Autodesk Inventor part; units mm, degrees
(part 2 of 3)
  spline S148 degree 2 poles (-84.7647, -63.9255) (-84.6572, -63.7642) (-84.2951, -63.5775) (-84.0744, -63.5775) knots 0 0 0 1 2 2 2
  spline S149 degree 2 poles (-84.0744, -63.5775) (-83.6641, -63.5775) (-83.2227, -64.1263) (-83.2227, -64.6554) knots 0 0 0 1 2 2 2
  spline S150 degree 2 poles (-84.1423, -64.6809) (-84.1423, -64.463) (-84.3092, -64.2423) (-84.4676, -64.2423) knots 0 0 0 1 2 2 2
  spline S151 degree 2 poles (-84.4676, -64.2423) (-84.6063, -64.2423) (-84.7902, -64.4743) (-84.7902, -64.6583) knots 0 0 0 1 2 2 2
  line L119 (-84.7902, -64.6583) -> (-84.7902, -64.7912)
  spline S152 degree 2 poles (-84.7902, -64.7912) (-84.7902, -64.978) (-84.6233, -65.1987) (-84.4846, -65.1987) knots 0 0 0 1 2 2 2
  spline S153 degree 2 poles (-84.4846, -65.1987) (-84.3205, -65.1987) (-84.1423, -64.9299) (-84.1423, -64.6809) knots 0 0 0 1 2 2 2
  spline S154 degree 2 poles (-82.4588, -66.834) (-82.5862, -66.834) (-82.8776, -66.7887) (-82.9936, -66.7463) knots 0 0 0 1 2 2 2
  line L120 (-82.9936, -66.7463) -> (-82.9936, -66.0644)
  spline S155 degree 2 poles (-82.9936, -66.0644) (-82.9398, -66.104) (-82.7304, -66.1719) (-82.6371, -66.1719) knots 0 0 0 1 2 2 2
  spline S156 degree 2 poles (-82.6371, -66.1719) (-82.3824, -66.1719) (-82.3004, -65.9711) knots 0 0 0 1 1 1
  line L121 (-82.3004, -65.9711) -> (-82.2297, -65.8013)
  line L122 (-82.2297, -65.8013) -> (-83.1407, -63.6312)
  line L123 (-83.1407, -63.6312) -> (-82.1391, -63.6312)
  line L124 (-82.1391, -63.6312) -> (-81.876, -64.6809)
  spline S157 degree 2 poles (-81.876, -64.6809) (-81.7996, -64.9751) (-81.7911, -65.077) knots 0 0 0 1 1 1
  line L125 (-81.7911, -65.077) -> (-81.7826, -65.077)
  spline S158 degree 2 poles (-81.7826, -65.077) (-81.777, -65.0289) (-81.7543, -64.9157) (-81.4346, -63.6312) knots 0 0 0 1 2 2 2
  line L126 (-81.4346, -63.6312) -> (-80.5547, -63.6312)
  line L127 (-80.5547, -63.6312) -> (-81.3554, -65.872)
  spline S159 degree 2 poles (-81.3554, -65.872) (-81.5365, -66.387) (-82.0712, -66.834) (-82.4588, -66.834) knots 0 0 0 1 2 2 2
  spline S160 degree 2 poles (-79.3947, -65.4307) (-79.3947, -65.6259) (-79.6663, -65.8635) (-79.9068, -65.8635) knots 0 0 0 1 2 2 2
  spline S161 degree 2 poles (-79.9068, -65.8635) (-80.1275, -65.8635) (-80.4048, -65.6146) (-80.4048, -65.4307) knots 0 0 0 1 2 2 2
  spline S162 degree 2 poles (-80.4048, -65.4307) (-80.4048, -65.2439) (-80.1303, -65.0119) (-79.8983, -65.0119) knots 0 0 0 1 2 2 2
  spline S163 degree 2 poles (-79.8983, -65.0119) (-79.672, -65.0119) (-79.3947, -65.2439) (-79.3947, -65.4307) knots 0 0 0 1 2 2 2
  spline S164 degree 2 poles (-79.3947, -64.05) (-79.3947, -64.2452) (-79.6691, -64.48) (-79.9068, -64.48) knots 0 0 0 1 2 2 2
  spline S165 degree 2 poles (-79.9068, -64.48) (-80.1246, -64.48) (-80.4048, -64.2339) (-80.4048, -64.05) knots 0 0 0 1 2 2 2
  spline S166 degree 2 poles (-80.4048, -64.05) (-80.4048, -63.8632) (-80.1303, -63.6312) (-79.8983, -63.6312) knots 0 0 0 1 2 2 2
  spline S167 degree 2 poles (-79.8983, -63.6312) (-79.672, -63.6312) (-79.3947, -63.8632) (-79.3947, -64.05) knots 0 0 0 1 2 2 2
  spline S168 degree 2 poles (-137.9162, -70.7081) (-137.9162, -70.8722) (-138.086, -71.1636) (-138.3774, -71.3305) (-138.5387, -71.3305) knots 0 0 0 1 2 3 3 3
  spline S169 degree 2 poles (-138.5387, -71.3305) (-138.7905, -71.3305) (-139.1526, -70.9684) (-139.1526, -70.7081) knots 0 0 0 1 2 2 2
  spline S170 degree 2 poles (-139.1526, -70.7081) (-139.1526, -70.4563) (-138.7961, -70.0941) (-138.5387, -70.0941) knots 0 0 0 1 2 2 2
  spline S171 degree 2 poles (-138.5387, -70.0941) (-138.2755, -70.0941) (-137.9162, -70.4619) (-137.9162, -70.7081) knots 0 0 0 1 2 2 2
  line L128 (-128.1268, -71.7464) -> (-128.2598, -71.1862)
  line L129 (-128.2598, -71.1862) -> (-129.1708, -71.1862)
  line L130 (-129.1708, -71.1862) -> (-129.3151, -71.7464)
  line L131 (-129.3151, -71.7464) -> (-130.3082, -71.7464)
  line L132 (-130.3082, -71.7464) -> (-129.2585, -68.6964)
  line L133 (-129.2585, -68.6964) -> (-128.1183, -68.6964)
  line L134 (-128.1183, -68.6964) -> (-127.128, -71.7464)
  line L135 (-127.128, -71.7464) -> (-128.1268, -71.7464)
  line L136 (-128.704, -69.3613) -> (-128.7238, -69.3613)
  spline S172 degree 2 poles (-128.7238, -69.3613) (-128.7294, -69.4123) (-128.7804, -69.6471) (-129.0124, -70.5327) knots 0 0 0 1 2 2 2
  line L137 (-129.0124, -70.5327) -> (-128.4295, -70.5327)
  line L138 (-128.4295, -70.5327) -> (-128.6417, -69.7037)
  spline S173 degree 2 poles (-128.6417, -69.7037) (-128.687, -69.5198) (-128.704, -69.3613) knots 0 0 0 1 1 1
  line L139 (-126.8536, -71.7464) -> (-126.8536, -68.521)
  line L140 (-126.8536, -68.521) -> (-125.9482, -68.521)
  line L141 (-125.9482, -68.521) -> (-125.9482, -71.7464)
  line L142 (-125.9482, -71.7464) -> (-126.8536, -71.7464)
  spline S174 degree 2 poles (-123.8347, -69.1803) (-123.9762, -69.1322) (-124.095, -69.1322) knots 0 0 0 1 1 1
  spline S175 degree 2 poles (-124.095, -69.1322) (-124.2478, -69.1322) (-124.3921, -69.2878) (-124.3921, -69.4179) knots 0 0 0 1 2 2 2
  line L143 (-124.3921, -69.4179) -> (-124.3921, -69.5679)
  line L144 (-124.3921, -69.5679) -> (-123.8885, -69.5679)
  line L145 (-123.8885, -69.5679) -> (-123.8885, -70.196)
  line L146 (-123.8885, -70.196) -> (-124.3921, -70.196)
  line L147 (-124.3921, -70.196) -> (-124.3921, -71.7464)
  line L148 (-124.3921, -71.7464) -> (-125.2975, -71.7464)
  line L149 (-125.2975, -71.7464) -> (-125.2975, -70.196)
  line L150 (-125.2975, -70.196) -> (-125.6625, -70.196)
  line L151 (-125.6625, -70.196) -> (-125.6625, -69.5679)
  line L152 (-125.6625, -69.5679) -> (-125.2975, -69.5679)
  line L153 (-125.2975, -69.5679) -> (-125.2975, -69.367)
  spline S176 degree 2 poles (-125.2975, -69.367) (-125.2975, -69.101) (-125.0513, -68.6964) (-124.5817, -68.4701) (-124.245, -68.4701) knots 0 0 0 1 2 3 3 3
  spline S177 degree 2 poles (-124.245, -68.4701) (-124.0016, -68.4701) (-123.8347, -68.5182) knots 0 0 0 1 1 1
  line L154 (-123.8347, -68.5182) -> (-123.8347, -69.1803)
  line L155 (-122.4257, -71.7464) -> (-122.4257, -71.4154)
  line L156 (-122.4257, -71.4154) -> (-122.4342, -71.4154)
  spline S178 degree 2 poles (-122.4342, -71.4154) (-122.6521, -71.8002) (-123.0991, -71.8002) knots 0 0 0 1 1 1
  spline S179 degree 2 poles (-123.0991, -71.8002) (-123.4075, -71.8002) (-123.7555, -71.4352) (-123.7555, -71.1268) knots 0 0 0 1 2 2 2
  spline S180 degree 2 poles (-123.7555, -71.1268) (-123.7555, -70.4846) (-122.9661, -70.3827) knots 0 0 0 1 1 1
  line L157 (-122.9661, -70.3827) -> (-122.4257, -70.312)
  spline S181 degree 2 poles (-122.4257, -70.312) (-122.4257, -70.2045) (-122.6181, -70.0687) (-122.7794, -70.0687) knots 0 0 0 1 2 2 2
  spline S182 degree 2 poles (-122.7794, -70.0687) (-123.1444, -70.0687) (-123.5518, -70.278) knots 0 0 0 1 1 1
  line L158 (-123.5518, -70.278) -> (-123.5518, -69.6895)
  spline S183 degree 2 poles (-123.5518, -69.6895) (-123.3764, -69.6131) (-122.8416, -69.5141) (-122.6521, -69.5141) knots 0 0 0 1 2 2 2
  spline S184 degree 2 poles (-122.6521, -69.5141) (-122.0975, -69.5141) (-121.5967, -69.9894) (-121.5967, -70.544) knots 0 0 0 1 2 2 2
  line L159 (-121.5967, -70.544) -> (-121.5967, -71.7464)
  line L160 (-121.5967, -71.7464) -> (-122.4257, -71.7464)
  spline S185 degree 2 poles (-122.9633, -71.0052) (-122.9633, -71.0929) (-122.8501, -71.2089) (-122.7454, -71.2089) knots 0 0 0 1 2 2 2
  spline S186 degree 2 poles (-122.7454, -71.2089) (-122.604, -71.2089) (-122.4257, -70.9967) (-122.4257, -70.8298) knots 0 0 0 1 2 2 2
  line L161 (-122.4257, -70.8298) -> (-122.4257, -70.7477)
  line L162 (-122.4257, -70.7477) -> (-122.7341, -70.7901)
  spline S187 degree 2 poles (-122.7341, -70.7901) (-122.9633, -70.8298) (-122.9633, -71.0052) knots 0 0 0 1 1 1
  line L163 (-119.7775, -71.7464) -> (-119.7775, -70.5581)
  spline S188 degree 2 poles (-119.7775, -70.5581) (-119.7775, -70.3544) (-119.8991, -70.179) (-120.0349, -70.179) knots 0 0 0 1 2 2 2
  spline S189 degree 2 poles (-120.0349, -70.179) (-120.1509, -70.179) (-120.2839, -70.3629) (-120.2839, -70.5044) knots 0 0 0 1 2 2 2
  line L164 (-120.2839, -70.5044) -> (-120.2839, -71.7464)
  line L165 (-120.2839, -71.7464) -> (-121.1893, -71.7464)
  line L166 (-121.1893, -71.7464) -> (-121.1893, -69.5679)
  line L167 (-121.1893, -69.5679) -> (-120.2839, -69.5679)
  line L168 (-120.2839, -69.5679) -> (-120.2839, -69.9074)
  line L169 (-120.2839, -69.9074) -> (-120.2754, -69.9074)
  spline S190 degree 2 poles (-120.2754, -69.9074) (-120.1679, -69.7207) (-119.8001, -69.5141) (-119.5851, -69.5141) knots 0 0 0 1 2 2 2
  spline S191 degree 2 poles (-119.5851, -69.5141) (-118.8721, -69.5141) (-118.8721, -70.4167) knots 0 0 0 1 1 1
  line L170 (-118.8721, -70.4167) -> (-118.8721, -71.7464)
  line L171 (-118.8721, -71.7464) -> (-119.7775, -71.7464)
  spline S192 degree 2 poles (-116.04, -70.6176) (-116.04, -71.1693) (-116.7048, -71.8002) (-117.3018, -71.8002) knots 0 0 0 1 2 2 2
  spline S193 degree 2 poles (-117.3018, -71.8002) (-117.896, -71.8002) (-118.558, -71.1862) (-118.558, -70.643) knots 0 0 0 1 2 2 2
  spline S194 degree 2 poles (-118.558, -70.643) (-118.558, -70.2978) (-118.2468, -69.7857) (-117.6725, -69.5141) (-117.299, -69.5141) knots 0 0 0 1 2 3 3 3
  spline S195 degree 2 poles (-117.299, -69.5141) (-116.9114, -69.5141) (-116.3427, -69.7999) (-116.04, -70.3063) (-116.04, -70.6176) knots 0 0 0 1 2 3 3 3
  spline S196 degree 2 poles (-116.9595, -70.6232) (-116.9595, -70.179) (-117.299, -70.179) knots 0 0 0 1 1 1
  spline S197 degree 2 poles (-117.299, -70.179) (-117.6385, -70.179) (-117.6385, -70.643) knots 0 0 0 1 1 1
  spline S198 degree 2 poles (-117.6385, -70.643) (-117.6385, -71.1353) (-117.2933, -71.1353) knots 0 0 0 1 1 1
  spline S199 degree 2 poles (-117.2933, -71.1353) (-116.9595, -71.1353) (-116.9595, -70.6232) knots 0 0 0 1 1 1
  line L172 (-114.4074, -71.7464) -> (-114.4074, -68.6964)
  line L173 (-114.4074, -68.6964) -> (-112.509, -68.6964)
  line L174 (-112.509, -68.6964) -> (-112.509, -69.4151)
  line L175 (-112.509, -69.4151) -> (-113.4879, -69.4151)
  line L176 (-113.4879, -69.4151) -> (-113.4879, -69.8593)
  line L177 (-113.4879, -69.8593) -> (-112.5684, -69.8593)
  line L178 (-112.5684, -69.8593) -> (-112.5684, -70.5779)
  line L179 (-112.5684, -70.5779) -> (-113.4879, -70.5779)
  line L180 (-113.4879, -70.5779) -> (-113.4879, -71.0278)
  line L181 (-113.4879, -71.0278) -> (-112.4382, -71.0278)
  line L182 (-112.4382, -71.0278) -> (-112.4382, -71.7464)
  line L183 (-112.4382, -71.7464) -> (-114.4074, -71.7464)
  line L184 (-109.2609, -71.7464) -> (-109.2609, -70.4902)
  spline S200 degree 2 poles (-109.2609, -70.4902) (-109.2609, -70.3346) (-109.3741, -70.179) (-109.5014, -70.179) knots 0 0 0 1 2 2 2
  spline S201 degree 2 poles (-109.5014, -70.179) (-109.6259, -70.179) (-109.7674, -70.3686) (-109.7674, -70.5355) knots 0 0 0 1 2 2 2
  line L185 (-109.7674, -70.5355) -> (-109.7674, -71.7464)
  line L186 (-109.7674, -71.7464) -> (-110.6727, -71.7464)
  line L187 (-110.6727, -71.7464) -> (-110.6727, -70.5129)
  spline S202 degree 2 poles (-110.6727, -70.5129) (-110.6727, -70.179) (-110.8991, -70.179) knots 0 0 0 1 1 1
  spline S203 degree 2 poles (-110.8991, -70.179) (-111.0377, -70.179) (-111.1792, -70.3714) (-111.1792, -70.5525) knots 0 0 0 1 2 2 2
  line L188 (-111.1792, -70.5525) -> (-111.1792, -71.7464)
  line L189 (-111.1792, -71.7464) -> (-112.0846, -71.7464)
  line L190 (-112.0846, -71.7464) -> (-112.0846, -69.5679)
  line L191 (-112.0846, -69.5679) -> (-111.1792, -69.5679)
  line L192 (-111.1792, -69.5679) -> (-111.1792, -69.9131)
  line L193 (-111.1792, -69.9131) -> (-111.1707, -69.9131)
  spline S204 degree 2 poles (-111.1707, -69.9131) (-111.1198, -69.8225) (-110.8963, -69.6301) (-110.6162, -69.5141) (-110.4521, -69.5141) knots 0 0 0 1 2 3 3 3
  spline S205 degree 2 poles (-110.4521, -69.5141) (-110.2201, -69.5141) (-109.9032, -69.698) (-109.7985, -69.8961) knots 0 0 0 1 2 2 2
  spline S206 degree 2 poles (-109.7985, -69.8961) (-109.6825, -69.7122) (-109.2977, -69.5141) (-109.0657, -69.5141) knots 0 0 0 1 2 2 2
  spline S207 degree 2 poles (-109.0657, -69.5141) (-108.7205, -69.5141) (-108.3555, -69.9612) (-108.3555, -70.3827) knots 0 0 0 1 2 2 2
  line L194 (-108.3555, -70.3827) -> (-108.3555, -71.7464)
  line L195 (-108.3555, -71.7464) -> (-109.2609, -71.7464)
  line L196 (-106.7372, -71.7464) -> (-106.7372, -71.4154)
  line L197 (-106.7372, -71.4154) -> (-106.7457, -71.4154)
  spline S208 degree 2 poles (-106.7457, -71.4154) (-106.9635, -71.8002) (-107.4106, -71.8002) knots 0 0 0 1 1 1
  spline S209 degree 2 poles (-107.4106, -71.8002) (-107.7189, -71.8002) (-108.067, -71.4352) (-108.067, -71.1268) knots 0 0 0 1 2 2 2
  spline S210 degree 2 poles (-108.067, -71.1268) (-108.067, -70.4846) (-107.2776, -70.3827) knots 0 0 0 1 1 1
  line L198 (-107.2776, -70.3827) -> (-106.7372, -70.312)
  spline S211 degree 2 poles (-106.7372, -70.312) (-106.7372, -70.2045) (-106.9296, -70.0687) (-107.0908, -70.0687) knots 0 0 0 1 2 2 2
  spline S212 degree 2 poles (-107.0908, -70.0687) (-107.4558, -70.0687) (-107.8632, -70.278) knots 0 0 0 1 1 1
  line L199 (-107.8632, -70.278) -> (-107.8632, -69.6895)
  spline S213 degree 2 poles (-107.8632, -69.6895) (-107.6878, -69.6131) (-107.1531, -69.5141) (-106.9635, -69.5141) knots 0 0 0 1 2 2 2
  spline S214 degree 2 poles (-106.9635, -69.5141) (-106.409, -69.5141) (-105.9082, -69.9894) (-105.9082, -70.544) knots 0 0 0 1 2 2 2
  line L200 (-105.9082, -70.544) -> (-105.9082, -71.7464)
  line L201 (-105.9082, -71.7464) -> (-106.7372, -71.7464)
  spline S215 degree 2 poles (-107.2747, -71.0052) (-107.2747, -71.0929) (-107.1616, -71.2089) (-107.0569, -71.2089) knots 0 0 0 1 2 2 2
  spline S216 degree 2 poles (-107.0569, -71.2089) (-106.9154, -71.2089) (-106.7372, -70.9967) (-106.7372, -70.8298) knots 0 0 0 1 2 2 2
  line L202 (-106.7372, -70.8298) -> (-106.7372, -70.7477)
  line L203 (-106.7372, -70.7477) -> (-107.0456, -70.7901)
  spline S217 degree 2 poles (-107.0456, -70.7901) (-107.2747, -70.8298) (-107.2747, -71.0052) knots 0 0 0 1 1 1
  line L204 (-104.0889, -71.7464) -> (-104.0889, -70.5581)
  spline S218 degree 2 poles (-104.0889, -70.5581) (-104.0889, -70.3544) (-104.2106, -70.179) (-104.3464, -70.179) knots 0 0 0 1 2 2 2
  spline S219 degree 2 poles (-104.3464, -70.179) (-104.4624, -70.179) (-104.5954, -70.3629) (-104.5954, -70.5044) knots 0 0 0 1 2 2 2
  line L205 (-104.5954, -70.5044) -> (-104.5954, -71.7464)
  line L206 (-104.5954, -71.7464) -> (-105.5008, -71.7464)
  line L207 (-105.5008, -71.7464) -> (-105.5008, -69.5679)
  line L208 (-105.5008, -69.5679) -> (-104.5954, -69.5679)
  line L209 (-104.5954, -69.5679) -> (-104.5954, -69.9074)
  line L210 (-104.5954, -69.9074) -> (-104.5869, -69.9074)
  spline S220 degree 2 poles (-104.5869, -69.9074) (-104.4794, -69.7207) (-104.1116, -69.5141) (-103.8965, -69.5141) knots 0 0 0 1 2 2 2
  spline S221 degree 2 poles (-103.8965, -69.5141) (-103.1836, -69.5141) (-103.1836, -70.4167) knots 0 0 0 1 1 1
  line L211 (-103.1836, -70.4167) -> (-103.1836, -71.7464)
  line L212 (-103.1836, -71.7464) -> (-104.0889, -71.7464)
  line L213 (-101.3869, -71.7464) -> (-101.3869, -71.4098)
  line L214 (-101.3869, -71.4098) -> (-101.3954, -71.4098)
  spline S222 degree 2 poles (-101.3954, -71.4098) (-101.5086, -71.5654) (-101.6897, -71.7097) (-101.916, -71.8002) (-102.066, -71.8002) knots 0 0 0 1 2 3 3 3
  spline S223 degree 2 poles (-102.066, -71.8002) (-102.4253, -71.8002) (-102.7988, -71.3362) (-102.7988, -70.8835) knots 0 0 0 1 2 2 2
  line L215 (-102.7988, -70.8835) -> (-102.7988, -69.5679)
  line L216 (-102.7988, -69.5679) -> (-101.8934, -69.5679)
  line L217 (-101.8934, -69.5679) -> (-101.8934, -70.8128)
  spline S224 degree 2 poles (-101.8934, -70.8128) (-101.8934, -71.1353) (-101.6529, -71.1353) knots 0 0 0 1 1 1
  spline S225 degree 2 poles (-101.6529, -71.1353) (-101.5199, -71.1353) (-101.3869, -70.9599) (-101.3869, -70.8015) knots 0 0 0 1 2 2 2
  line L218 (-101.3869, -70.8015) -> (-101.3869, -69.5679)
  line L219 (-101.3869, -69.5679) -> (-100.4816, -69.5679)
  line L220 (-100.4816, -69.5679) -> (-100.4816, -71.7464)
  line L221 (-100.4816, -71.7464) -> (-101.3869, -71.7464)
  spline S226 degree 2 poles (-99.265, -70.9146) (-99.2423, -71.0561) (-98.965, -71.2145) (-98.7387, -71.2145) knots 0 0 0 1 2 2 2
  spline S227 degree 2 poles (-98.7387, -71.2145) (-98.4218, -71.2145) (-98.1389, -71.0929) knots 0 0 0 1 1 1
  line L222 (-98.1389, -71.0929) -> (-98.1389, -71.6672)
  spline S228 degree 2 poles (-98.1389, -71.6672) (-98.4671, -71.8002) (-98.9396, -71.8002) knots 0 0 0 1 1 1
  spline S229 degree 2 poles (-98.9396, -71.8002) (-99.5083, -71.8002) (-100.142, -71.2174) (-100.142, -70.7053) knots 0 0 0 1 2 2 2
  spline S230 degree 2 poles (-100.142, -70.7053) (-100.142, -70.3544) (-99.8648, -69.8197) (-99.3187, -69.5141) (-98.9877, -69.5141) knots 0 0 0 1 2 3 3 3
  spline S231 degree 2 poles (-98.9877, -69.5141) (-98.651, -69.5141) (-98.17, -69.7772) (-97.921, -70.2554) (-97.921, -70.5751) knots 0 0 0 1 2 3 3 3
  line L223 (-97.921, -70.5751) -> (-97.921, -70.9146)
  line L224 (-97.921, -70.9146) -> (-99.265, -70.9146)
  spline S232 degree 2 poles (-98.7217, -70.4393) (-98.7217, -70.063) (-98.9905, -70.063) knots 0 0 0 1 1 1
  spline S233 degree 2 poles (-98.9905, -70.063) (-99.1037, -70.063) (-99.2565, -70.2695) (-99.2706, -70.4393) knots 0 0 0 1 2 2 2
  line L225 (-99.2706, -70.4393) -> (-98.7217, -70.4393)
  line L226 (-97.607, -71.7464) -> (-97.607, -68.521)
  line L227 (-97.607, -68.521) -> (-96.7016, -68.521)
  line L228 (-96.7016, -68.521) -> (-96.7016, -71.7464)
  line L229 (-96.7016, -71.7464) -> (-97.607, -71.7464)
  spline S234 degree 2 poles (-95.485, -70.9146) (-95.4624, -71.0561) (-95.1851, -71.2145) (-94.9587, -71.2145) knots 0 0 0 1 2 2 2
  spline S235 degree 2 poles (-94.9587, -71.2145) (-94.6419, -71.2145) (-94.3589, -71.0929) knots 0 0 0 1 1 1
  line L230 (-94.3589, -71.0929) -> (-94.3589, -71.6672)
  spline S236 degree 2 poles (-94.3589, -71.6672) (-94.6871, -71.8002) (-95.1596, -71.8002) knots 0 0 0 1 1 1
  spline S237 degree 2 poles (-95.1596, -71.8002) (-95.7283, -71.8002) (-96.3621, -71.2174) (-96.3621, -70.7053) knots 0 0 0 1 2 2 2
  spline S238 degree 2 poles (-96.3621, -70.7053) (-96.3621, -70.3544) (-96.0848, -69.8197) (-95.5388, -69.5141) (-95.2077, -69.5141) knots 0 0 0 1 2 3 3 3
  spline S239 degree 2 poles (-95.2077, -69.5141) (-94.871, -69.5141) (-94.39, -69.7772) (-94.1411, -70.2554) (-94.1411, -70.5751) knots 0 0 0 1 2 3 3 3
  line L231 (-94.1411, -70.5751) -> (-94.1411, -70.9146)
  line L232 (-94.1411, -70.9146) -> (-95.485, -70.9146)
  spline S240 degree 2 poles (-94.9418, -70.4393) (-94.9418, -70.063) (-95.2106, -70.063) knots 0 0 0 1 1 1
  spline S241 degree 2 poles (-95.2106, -70.063) (-95.3237, -70.063) (-95.4765, -70.2695) (-95.4907, -70.4393) knots 0 0 0 1 2 2 2
  line L233 (-95.4907, -70.4393) -> (-94.9418, -70.4393)
  spline S242 degree 2 poles (-24.5942, -53.8935) (-24.5942, -54.289) (-24.8759, -55.0008) (-25.128, -55.248) knots 0 0 0 1 2 2 2
  spline S243 degree 2 poles (-25.128, -55.248) (-25.4444, -55.5594) (-26.2996, -55.8807) (-26.9521, -55.8807) knots 0 0 0 1 2 2 2
  line L234 (-26.9521, -55.8807) -> (-27.6392, -55.8807)
  line L235 (-27.6392, -55.8807) -> (-27.6392, -58.1546)
  line L236 (-27.6392, -58.1546) -> (-28.4499, -58.1546)
  line L237 (-28.4499, -58.1546) -> (-28.4499, -52.0546)
  line L238 (-28.4499, -52.0546) -> (-26.9175, -52.0546)
  spline S244 degree 2 poles (-26.9175, -52.0546) (-26.3737, -52.0546) (-25.6125, -52.2326) (-25.3208, -52.4353) knots 0 0 0 1 2 2 2
  spline S245 degree 2 poles (-25.3208, -52.4353) (-24.9797, -52.6676) (-24.5942, -53.3844) (-24.5942, -53.8935) knots 0 0 0 1 2 2 2
  spline S246 degree 2 poles (-25.4395, -53.9182) (-25.4395, -53.6019) (-25.657, -53.1372) (-25.8794, -52.9889) knots 0 0 0 1 2 2 2
  spline S247 degree 2 poles (-25.8794, -52.9889) (-26.0722, -52.8604) (-26.5863, -52.7566) (-26.9669, -52.7566) knots 0 0 0 1 2 2 2
  line L239 (-26.9669, -52.7566) -> (-27.6392, -52.7566)
  line L240 (-27.6392, -52.7566) -> (-27.6392, -55.1887)
  line L241 (-27.6392, -55.1887) -> (-27.0856, -55.1887)
  spline S248 degree 2 poles (-27.0856, -55.1887) (-26.5913, -55.1887) (-25.9832, -55.0305) (-25.7855, -54.8229) knots 0 0 0 1 2 2 2
  spline S249 degree 2 poles (-25.7855, -54.8229) (-25.6026, -54.64) (-25.4395, -54.2099) (-25.4395, -53.9182) knots 0 0 0 1 2 2 2
  line L242 (-21.4552, -54.4027) -> (-21.4947, -54.4027)
  spline S250 degree 2 poles (-21.4947, -54.4027) (-21.5837, -54.378) (-21.7765, -54.3681) (-21.91, -54.3681) knots 0 0 0 1 2 2 2
  spline S251 degree 2 poles (-21.91, -54.3681) (-22.2214, -54.3681) (-22.8344, -54.64) (-23.1112, -54.9069) knots 0 0 0 1 2 2 2
  line L243 (-23.1112, -54.9069) -> (-23.1112, -58.1546)
  line L244 (-23.1112, -58.1546) -> (-23.8823, -58.1546)
  line L245 (-23.8823, -58.1546) -> (-23.8823, -53.5772)
  line L246 (-23.8823, -53.5772) -> (-23.1112, -53.5772)
  line L247 (-23.1112, -53.5772) -> (-23.1112, -54.2593)
  spline S252 degree 2 poles (-23.1112, -54.2593) (-22.691, -53.8836) (-22.0632, -53.5772) (-21.7666, -53.5772) knots 0 0 0 1 2 2 2
  spline S253 degree 2 poles (-21.7666, -53.5772) (-21.648, -53.5772) (-21.5293, -53.587) (-21.4552, -53.6019) knots 0 0 0 1 2 2 2
  line L248 (-21.4552, -53.6019) -> (-21.4552, -54.4027)
  spline S254 degree 2 poles (-17.0952, -55.8659) (-17.0952, -57.0226) (-18.2075, -58.2832) (-19.1368, -58.2832) knots 0 0 0 1 2 2 2
  spline S255 degree 2 poles (-19.1368, -58.2832) (-20.0908, -58.2832) (-21.1833, -56.9831) (-21.1833, -55.8659) knots 0 0 0 1 2 2 2
  spline S256 degree 2 poles (-21.1833, -55.8659) (-21.1833, -54.7191) (-20.0562, -53.4486) (-19.1368, -53.4486) knots 0 0 0 1 2 2 2
  spline S257 degree 2 poles (-19.1368, -53.4486) (-18.2075, -53.4486) (-17.0952, -54.7141) (-17.0952, -55.8659) knots 0 0 0 1 2 2 2
  spline S258 degree 2 poles (-17.8911, -55.8659) (-17.8911, -54.9761) (-18.5387, -54.111) (-19.1368, -54.111) knots 0 0 0 1 2 2 2
  spline S259 degree 2 poles (-19.1368, -54.111) (-19.7349, -54.111) (-20.3874, -54.9761) (-20.3874, -55.8659) knots 0 0 0 1 2 2 2
  spline S260 degree 2 poles (-20.3874, -55.8659) (-20.3874, -56.731) (-19.7349, -57.6208) (-19.1368, -57.6208) knots 0 0 0 1 2 2 2
  spline S261 degree 2 poles (-19.1368, -57.6208) (-18.5436, -57.6208) (-17.8911, -56.7458) (-17.8911, -55.8659) knots 0 0 0 1 2 2 2
  spline S262 degree 2 poles (-16.1412, -58.8862) (-16.0621, -58.9208) (-15.7605, -59.0296) (-15.5677, -59.0741) knots 0 0 0 1 2 2 2
  spline S263 degree 2 poles (-15.5677, -59.0741) (-15.3552, -59.1285) (-14.9943, -59.1927) (-14.7818, -59.1927) knots 0 0 0 1 2 2 2
  spline S264 degree 2 poles (-14.7818, -59.1927) (-14.4259, -59.1927) (-13.9315, -59.0049) (-13.7931, -58.8368) knots 0 0 0 1 2 2 2
  spline S265 degree 2 poles (-13.7931, -58.8368) (-13.6596, -58.6687) (-13.5558, -58.2288) (-13.5558, -57.947) knots 0 0 0 1 2 2 2
  line L249 (-13.5558, -57.947) -> (-13.5558, -57.5466)
  spline S266 degree 2 poles (-13.5558, -57.5466) (-13.8673, -57.8185) (-14.4654, -58.0755) (-14.9152, -58.0755) knots 0 0 0 1 2 2 2
  spline S267 degree 2 poles (-14.9152, -58.0755) (-15.6963, -58.0755) (-16.6207, -56.9139) (-16.6207, -55.8214) knots 0 0 0 1 2 2 2
  spline S268 degree 2 poles (-16.6207, -55.8214) (-16.6207, -55.2529) (-16.2994, -54.373) (-16.0324, -54.0616) knots 0 0 0 1 2 2 2
  spline S269 degree 2 poles (-16.0324, -54.0616) (-15.7754, -53.7699) (-15.0685, -53.4486) (-14.6928, -53.4486) knots 0 0 0 1 2 2 2
  spline S270 degree 2 poles (-14.6928, -53.4486) (-14.3369, -53.4486) (-13.8178, -53.6167) (-13.5558, -53.7699) knots 0 0 0 1 2 2 2
  line L250 (-13.5558, -53.7699) -> (-13.5113, -53.5772)
  line L251 (-13.5113, -53.5772) -> (-12.7847, -53.5772)
  line L252 (-12.7847, -53.5772) -> (-12.7847, -57.6306)
  spline S271 degree 2 poles (-12.7847, -57.6306) (-12.7847, -58.7973) (-13.7981, -59.8848) (-14.8411, -59.8848) knots 0 0 0 1 2 2 2
  spline S272 degree 2 poles (-14.8411, -59.8848) (-15.1772, -59.8848) (-15.8792, -59.776) (-16.1807, -59.687) knots 0 0 0 1 2 2 2
  line L253 (-16.1807, -59.687) -> (-16.1807, -58.8862)
  line L254 (-16.1807, -58.8862) -> (-16.1412, -58.8862)
  line L255 (-13.5558, -56.9139) -> (-13.5558, -54.3977)
  spline S273 degree 2 poles (-13.5558, -54.3977) (-13.8425, -54.2593) (-14.327, -54.1407) (-14.5692, -54.1407) knots 0 0 0 1 2 2 2
  spline S274 degree 2 poles (-14.5692, -54.1407) (-15.1525, -54.1407) (-15.8248, -55.0008) (-15.8248, -55.8066) knots 0 0 0 1 2 2 2
  spline S275 degree 2 poles (-15.8248, -55.8066) (-15.8248, -56.5678) (-15.3156, -57.3637) (-14.7422, -57.3637) knots 0 0 0 1 2 2 2
  spline S276 degree 2 poles (-14.7422, -57.3637) (-14.4407, -57.3637) (-13.8079, -57.1264) (-13.5558, -56.9139) knots 0 0 0 1 2 2 2
  spline S277 degree 2 poles (-9.6803, -58.2584) (-10.7777, -58.2584) (-11.9839, -57.0276) (-11.9839, -55.8906) knots 0 0 0 1 2 2 2
  spline S278 degree 2 poles (-11.9839, -55.8906) (-11.9839, -54.7734) (-10.8123, -53.4486) (-9.8682, -53.4486) knots 0 0 0 1 2 2 2
  spline S279 degree 2 poles (-9.8682, -53.4486) (-9.443, -53.4486) (-8.7856, -53.6958) (-8.5434, -53.9578) knots 0 0 0 1 2 2 2
  spline S280 degree 2 poles (-8.5434, -53.9578) (-8.2962, -54.2198) (-8.0342, -54.9761) (-8.0342, -55.5248) knots 0 0 0 1 2 2 2
  line L256 (-8.0342, -55.5248) -> (-8.0342, -55.945)
  line L257 (-8.0342, -55.945) -> (-11.2028, -55.945)
  spline S281 degree 2 poles (-11.2028, -55.945) (-11.2028, -56.7409) (-10.402, -57.5862) (-9.6902, -57.5862) knots 0 0 0 1 2 2 2
  spline S282 degree 2 poles (-9.6902, -57.5862) (-9.4381, -57.5862) (-8.9487, -57.4725) (-8.751, -57.3835) knots 0 0 0 1 2 2 2
  spline S283 degree 2 poles (-8.751, -57.3835) (-8.5434, -57.2846) (-8.2566, -57.1116) (-8.1627, -57.0325) knots 0 0 0 1 2 2 2
  line L258 (-8.1627, -57.0325) -> (-8.1182, -57.0325)
  line L259 (-8.1182, -57.0325) -> (-8.1182, -57.8729)
  spline S284 degree 2 poles (-8.1182, -57.8729) (-8.2517, -57.9272) (-8.6571, -58.0854) (-8.8152, -58.1299) knots 0 0 0 1 2 2 2
  spline S285 degree 2 poles (-8.8152, -58.1299) (-9.0377, -58.1942) (-9.4035, -58.2584) (-9.6803, -58.2584) knots 0 0 0 1 2 2 2
  spline S286 degree 2 poles (-8.7856, -55.3567) (-8.7955, -55.0453) (-8.924, -54.5905) (-9.0476, -54.4373) knots 0 0 0 1 2 2 2
  spline S287 degree 2 poles (-9.0476, -54.4373) (-9.181, -54.2643) (-9.6012, -54.0814) (-9.9126, -54.0814) knots 0 0 0 1 2 2 2
  spline S288 degree 2 poles (-9.9126, -54.0814) (-10.2191, -54.0814) (-10.6492, -54.2643) (-10.8272, -54.4422) knots 0 0 0 1 2 2 2
  spline S289 degree 2 poles (-10.8272, -54.4422) (-11.0002, -54.6251) (-11.1781, -55.0651) (-11.2028, -55.3567) knots 0 0 0 1 2 2 2
  line L260 (-11.2028, -55.3567) -> (-8.7856, -55.3567)
  spline S290 degree 2 poles (-5.869, -58.2436) (-6.4968, -58.2436) (-7.2037, -57.5268) (-7.2037, -56.7507) knots 0 0 0 1 2 2 2
  line L261 (-7.2037, -56.7507) -> (-7.2037, -54.2148)
  line L262 (-7.2037, -54.2148) -> (-7.7228, -54.2148)
  line L263 (-7.7228, -54.2148) -> (-7.7228, -53.5772)
  line L264 (-7.7228, -53.5772) -> (-7.2037, -53.5772)
  line L265 (-7.2037, -53.5772) -> (-7.2037, -52.2622)
  line L266 (-7.2037, -52.2622) -> (-6.4326, -52.2622)
  line L267 (-6.4326, -52.2622) -> (-6.4326, -53.5772)
  line L268 (-6.4326, -53.5772) -> (-5.0139, -53.5772)
  line L269 (-5.0139, -53.5772) -> (-5.0139, -54.2148)
  line L270 (-5.0139, -54.2148) -> (-6.4326, -54.2148)
  line L271 (-6.4326, -54.2148) -> (-6.4326, -56.3948)
  spline S291 degree 2 poles (-6.4326, -56.3948) (-6.4326, -56.7409) (-6.4079, -57.1215) (-6.3238, -57.2846) knots 0 0 0 1 2 2 2
  spline S292 degree 2 poles (-6.3238, -57.2846) (-6.2546, -57.428) (-5.9432, -57.5713) (-5.6763, -57.5713) knots 0 0 0 1 2 2 2
  spline S293 degree 2 poles (-5.6763, -57.5713) (-5.4884, -57.5713) (-5.1374, -57.4576) (-5.0583, -57.423) knots 0 0 0 1 2 2 2
  line L272 (-5.0583, -57.423) -> (-5.0139, -57.423)
  line L273 (-5.0139, -57.423) -> (-5.0139, -58.1151)
  spline S294 degree 2 poles (-5.0139, -58.1151) (-5.2314, -58.1744) (-5.6763, -58.2436) (-5.869, -58.2436) knots 0 0 0 1 2 2 2
  spline S295 degree 2 poles (-3.0613, -58.2436) (-3.6891, -58.2436) (-4.396, -57.5268) (-4.396, -56.7507) knots 0 0 0 1 2 2 2
  line L274 (-4.396, -56.7507) -> (-4.396, -54.2148)
  line L275 (-4.396, -54.2148) -> (-4.915, -54.2148)
  line L276 (-4.915, -54.2148) -> (-4.915, -53.5772)
  line L277 (-4.915, -53.5772) -> (-4.396, -53.5772)
  line L278 (-4.396, -53.5772) -> (-4.396, -52.2622)
  line L279 (-4.396, -52.2622) -> (-3.6248, -52.2622)
  line L280 (-3.6248, -52.2622) -> (-3.6248, -53.5772)
  line L281 (-3.6248, -53.5772) -> (-2.2061, -53.5772)
  line L282 (-2.2061, -53.5772) -> (-2.2061, -54.2148)
  line L283 (-2.2061, -54.2148) -> (-3.6248, -54.2148)
  line L284 (-3.6248, -54.2148) -> (-3.6248, -56.3948)
  spline S296 degree 2 poles (-3.6248, -56.3948) (-3.6248, -56.7409) (-3.6001, -57.1215) (-3.516, -57.2846) knots 0 0 0 1 2 2 2
  spline S297 degree 2 poles (-3.516, -57.2846) (-3.4468, -57.428) (-3.1354, -57.5713) (-2.8685, -57.5713) knots 0 0 0 1 2 2 2
  spline S298 degree 2 poles (-2.8685, -57.5713) (-2.6806, -57.5713) (-2.3297, -57.4576) (-2.2506, -57.423) knots 0 0 0 1 2 2 2
  line L285 (-2.2506, -57.423) -> (-2.2061, -57.423)
  line L286 (-2.2061, -57.423) -> (-2.2061, -58.1151)
  spline S299 degree 2 poles (-2.2061, -58.1151) (-2.4236, -58.1744) (-2.8685, -58.2436) (-3.0613, -58.2436) knots 0 0 0 1 2 2 2
  spline S300 degree 2 poles (2.1242, -55.8659) (2.1242, -57.0226) (1.012, -58.2832) (0.0827, -58.2832) knots 0 0 0 1 2 2 2
  spline S301 degree 2 poles (0.0827, -58.2832) (-0.8714, -58.2832) (-1.9639, -56.9831) (-1.9639, -55.8659) knots 0 0 0 1 2 2 2
  spline S302 degree 2 poles (-1.9639, -55.8659) (-1.9639, -54.7191) (-0.8368, -53.4486) (0.0827, -53.4486) knots 0 0 0 1 2 2 2
  spline S303 degree 2 poles (0.0827, -53.4486) (1.012, -53.4486) (2.1242, -54.7141) (2.1242, -55.8659) knots 0 0 0 1 2 2 2
  spline S304 degree 2 poles (1.3284, -55.8659) (1.3284, -54.9761) (0.6808, -54.111) (0.0827, -54.111) knots 0 0 0 1 2 2 2
  spline S305 degree 2 poles (0.0827, -54.111) (-0.5155, -54.111) (-1.168, -54.9761) (-1.168, -55.8659) knots 0 0 0 1 2 2 2
  spline S306 degree 2 poles (-1.168, -55.8659) (-1.168, -56.731) (-0.5155, -57.6208) (0.0827, -57.6208) knots 0 0 0 1 2 2 2
  spline S307 degree 2 poles (0.0827, -57.6208) (0.6758, -57.6208) (1.3284, -56.7458) (1.3284, -55.8659) knots 0 0 0 1 2 2 2
  spline S308 degree 2 poles (7.9771, -58.2634) (7.3839, -58.2634) (6.3804, -57.863) (6.0146, -57.4626) knots 0 0 0 1 2 2 2
  spline S309 degree 2 poles (6.0146, -57.4626) (5.6488, -57.0671) (5.2484, -55.8807) (5.2484, -55.1096) knots 0 0 0 1 2 2 2
  spline S310 degree 2 poles (5.2484, -55.1096) (5.2484, -54.3434) (5.6389, -53.2064) (6.0096, -52.7862) knots 0 0 0 1 2 2 2
  spline S311 degree 2 poles (6.0096, -52.7862) (6.3754, -52.3759) (7.374, -51.9459) (7.9919, -51.9459) knots 0 0 0 1 2 2 2
  spline S312 degree 2 poles (7.9919, -51.9459) (8.2984, -51.9459) (8.8372, -52.0349) (9.0646, -52.1041) knots 0 0 0 1 2 2 2
  spline S313 degree 2 poles (9.0646, -52.1041) (9.2623, -52.1683) (9.6726, -52.3512) (9.8753, -52.46) knots 0 0 0 1 2 2 2
  line L287 (9.8753, -52.46) -> (9.8753, -53.4387)
  line L288 (9.8753, -53.4387) -> (9.811, -53.4387)
  spline S314 degree 2 poles (9.811, -53.4387) (9.7023, -53.3399) (9.3661, -53.0631) (9.1239, -52.9296) knots 0 0 0 1 2 2 2
  spline S315 degree 2 poles (9.1239, -52.9296) (8.8916, -52.8011) (8.3429, -52.6379) (7.987, -52.6379) knots 0 0 0 1 2 2 2
  spline S316 degree 2 poles (7.987, -52.6379) (7.5964, -52.6379) (6.8994, -52.9592) (6.6374, -53.2657) knots 0 0 0 1 2 2 2
  spline S317 degree 2 poles (6.6374, -53.2657) (6.3804, -53.5772) (6.0937, -54.5213) (6.0937, -55.1096) knots 0 0 0 1 2 2 2
  spline S318 degree 2 poles (6.0937, -55.1096) (6.0937, -55.7374) (6.3952, -56.642) (6.6572, -56.9534) knots 0 0 0 1 2 2 2
  spline S319 degree 2 poles (6.6572, -56.9534) (6.9143, -57.255) (7.6014, -57.5614) (7.987, -57.5614) knots 0 0 0 1 2 2 2
  spline S320 degree 2 poles (7.987, -57.5614) (8.3379, -57.5614) (8.9361, -57.3884) (9.1684, -57.2599) knots 0 0 0 1 2 2 2
  spline S321 degree 2 poles (9.1684, -57.2599) (9.3908, -57.1314) (9.722, -56.8644) (9.816, -56.7705) knots 0 0 0 1 2 2 2
  line L289 (9.816, -56.7705) -> (9.8753, -56.7705)
  line L290 (9.8753, -56.7705) -> (9.8753, -57.7394)
  spline S322 degree 2 poles (9.8753, -57.7394) (9.6726, -57.8333) (9.3167, -58.0063) (9.0646, -58.0854) knots 0 0 0 1 2 2 2
  spline S323 degree 2 poles (9.0646, -58.0854) (8.7976, -58.1744) (8.3429, -58.2634) (7.9771, -58.2634) knots 0 0 0 1 2 2 2
  spline S324 degree 2 poles (14.3341, -55.8659) (14.3341, -57.0226) (13.2219, -58.2832) (12.2925, -58.2832) knots 0 0 0 1 2 2 2
  spline S325 degree 2 poles (12.2925, -58.2832) (11.3385, -58.2832) (10.246, -56.9831) (10.246, -55.8659) knots 0 0 0 1 2 2 2
  spline S326 degree 2 poles (10.246, -55.8659) (10.246, -54.7191) (11.3731, -53.4486) (12.2925, -53.4486) knots 0 0 0 1 2 2 2
  spline S327 degree 2 poles (12.2925, -53.4486) (13.2219, -53.4486) (14.3341, -54.7141) (14.3341, -55.8659) knots 0 0 0 1 2 2 2
  spline S328 degree 2 poles (13.5382, -55.8659) (13.5382, -54.9761) (12.8907, -54.111) (12.2925, -54.111) knots 0 0 0 1 2 2 2
  spline S329 degree 2 poles (12.2925, -54.111) (11.6944, -54.111) (11.0419, -54.9761) (11.0419, -55.8659) knots 0 0 0 1 2 2 2
  spline S330 degree 2 poles (11.0419, -55.8659) (11.0419, -56.731) (11.6944, -57.6208) (12.2925, -57.6208) knots 0 0 0 1 2 2 2
  spline S331 degree 2 poles (12.2925, -57.6208) (12.8857, -57.6208) (13.5382, -56.7458) (13.5382, -55.8659) knots 0 0 0 1 2 2 2
  line L291 (18.7188, -58.1546) -> (17.9476, -58.1546)
  line L292 (17.9476, -58.1546) -> (17.9476, -55.5446)
  spline S332 degree 2 poles (17.9476, -55.5446) (17.9476, -55.2282) (17.8883, -54.6844) (17.7993, -54.5213) knots 0 0 0 1 2 2 2
  spline S333 degree 2 poles (17.7993, -54.5213) (17.7054, -54.3483) (17.3693, -54.1802) (17.0826, -54.1802) knots 0 0 0 1 2 2 2
  spline S334 degree 2 poles (17.0826, -54.1802) (16.7959, -54.1802) (16.1878, -54.4867) (15.8962, -54.7339) knots 0 0 0 1 2 2 2
  line L293 (15.8962, -54.7339) -> (15.8962, -58.1546)
  line L294 (15.8962, -58.1546) -> (15.125, -58.1546)
  line L295 (15.125, -58.1546) -> (15.125, -53.5772)
  line L296 (15.125, -53.5772) -> (15.8962, -53.5772)
  line L297 (15.8962, -53.5772) -> (15.8962, -54.0863)
  spline S335 degree 2 poles (15.8962, -54.0863) (16.2422, -53.7749) (16.9096, -53.4486) (17.2852, -53.4486) knots 0 0 0 1 2 2 2
  spline S336 degree 2 poles (17.2852, -53.4486) (17.9575, -53.4486) (18.7188, -54.3384) (18.7188, -55.1837) knots 0 0 0 1 2 2 2
  line L298 (18.7188, -55.1837) -> (18.7188, -58.1546)
  spline S337 degree 2 poles (21.1855, -58.2436) (20.5577, -58.2436) (19.8508, -57.5268) (19.8508, -56.7507) knots 0 0 0 1 2 2 2
  line L299 (19.8508, -56.7507) -> (19.8508, -54.2148)
  line L300 (19.8508, -54.2148) -> (19.3318, -54.2148)
  line L301 (19.3318, -54.2148) -> (19.3318, -53.5772)
  line L302 (19.3318, -53.5772) -> (19.8508, -53.5772)
  line L303 (19.8508, -53.5772) -> (19.8508, -52.2622)
  line L304 (19.8508, -52.2622) -> (20.622, -52.2622)
  line L305 (20.622, -52.2622) -> (20.622, -53.5772)
  line L306 (20.622, -53.5772) -> (22.0407, -53.5772)
  line L307 (22.0407, -53.5772) -> (22.0407, -54.2148)
  line L308 (22.0407, -54.2148) -> (20.622, -54.2148)
  line L309 (20.622, -54.2148) -> (20.622, -56.3948)
  spline S338 degree 2 poles (20.622, -56.3948) (20.622, -56.7409) (20.6467, -57.1215) (20.7307, -57.2846) knots 0 0 0 1 2 2 2
  spline S339 degree 2 poles (20.7307, -57.2846) (20.7999, -57.428) (21.1113, -57.5713) (21.3783, -57.5713) knots 0 0 0 1 2 2 2
  spline S340 degree 2 poles (21.3783, -57.5713) (21.5661, -57.5713) (21.9171, -57.4576) (21.9962, -57.423) knots 0 0 0 1 2 2 2
  line L310 (21.9962, -57.423) -> (22.0407, -57.423)
  line L311 (22.0407, -57.423) -> (22.0407, -58.1151)
  spline S341 degree 2 poles (22.0407, -58.1151) (21.8232, -58.1744) (21.3783, -58.2436) (21.1855, -58.2436) knots 0 0 0 1 2 2 2
  line L312 (25.0363, -54.4027) -> (24.9968, -54.4027)
  spline S342 degree 2 poles (24.9968, -54.4027) (24.9078, -54.378) (24.715, -54.3681) (24.5815, -54.3681) knots 0 0 0 1 2 2 2
  spline S343 degree 2 poles (24.5815, -54.3681) (24.2701, -54.3681) (23.6571, -54.64) (23.3803, -54.9069) knots 0 0 0 1 2 2 2
  line L313 (23.3803, -54.9069) -> (23.3803, -58.1546)
  line L314 (23.3803, -58.1546) -> (22.6092, -58.1546)
  line L315 (22.6092, -58.1546) -> (22.6092, -53.5772)
  line L316 (22.6092, -53.5772) -> (23.3803, -53.5772)
  line L317 (23.3803, -53.5772) -> (23.3803, -54.2593)
  spline S344 degree 2 poles (23.3803, -54.2593) (23.8005, -53.8836) (24.4283, -53.5772) (24.7249, -53.5772) knots 0 0 0 1 2 2 2
  spline S345 degree 2 poles (24.7249, -53.5772) (24.8435, -53.5772) (24.9622, -53.587) (25.0363, -53.6019) knots 0 0 0 1 2 2 2
  line L318 (25.0363, -53.6019) -> (25.0363, -54.4027)
  spline S346 degree 2 poles (29.3963, -55.8659) (29.3963, -57.0226) (28.284, -58.2832) (27.3547, -58.2832) knots 0 0 0 1 2 2 2
  spline S347 degree 2 poles (27.3547, -58.2832) (26.4006, -58.2832) (25.3082, -56.9831) (25.3082, -55.8659) knots 0 0 0 1 2 2 2
  spline S348 degree 2 poles (25.3082, -55.8659) (25.3082, -54.7191) (26.4352, -53.4486) (27.3547, -53.4486) knots 0 0 0 1 2 2 2
  spline S349 degree 2 poles (27.3547, -53.4486) (28.284, -53.4486) (29.3963, -54.7141) (29.3963, -55.8659) knots 0 0 0 1 2 2 2
  spline S350 degree 2 poles (28.6004, -55.8659) (28.6004, -54.9761) (27.9528, -54.111) (27.3547, -54.111) knots 0 0 0 1 2 2 2
  spline S351 degree 2 poles (27.3547, -54.111) (26.7566, -54.111) (26.1041, -54.9761) (26.1041, -55.8659) knots 0 0 0 1 2 2 2
  spline S352 degree 2 poles (26.1041, -55.8659) (26.1041, -56.731) (26.7566, -57.6208) (27.3547, -57.6208) knots 0 0 0 1 2 2 2
  spline S353 degree 2 poles (27.3547, -57.6208) (27.9479, -57.6208) (28.6004, -56.7458) (28.6004, -55.8659) knots 0 0 0 1 2 2 2
  line L319 (30.9732, -58.1546) -> (30.202, -58.1546)
  line L320 (30.202, -58.1546) -> (30.202, -51.7827)
  line L321 (30.202, -51.7827) -> (30.9732, -51.7827)
  line L322 (30.9732, -51.7827) -> (30.9732, -58.1546)
  line L323 (32.8912, -58.1546) -> (32.12, -58.1546)
  line L324 (32.12, -58.1546) -> (32.12, -51.7827)
  line L325 (32.12, -51.7827) -> (32.8912, -51.7827)
  line L326 (32.8912, -51.7827) -> (32.8912, -58.1546)
  line L327 (34.8092, -58.1546) -> (34.038, -58.1546)
  line L328 (34.038, -58.1546) -> (34.038, -53.5772)
  line L329 (34.038, -53.5772) -> (34.8092, -53.5772)
  line L330 (34.8092, -53.5772) -> (34.8092, -58.1546)
  line L331 (34.8635, -52.8159) -> (33.9886, -52.8159)
  line L332 (33.9886, -52.8159) -> (33.9886, -52.0151)
  line L333 (33.9886, -52.0151) -> (34.8635, -52.0151)
  line L334 (34.8635, -52.0151) -> (34.8635, -52.8159)
  line L335 (37.963, -58.1546) -> (40.0194, -52.0546)
  line L336 (40.0194, -52.0546) -> (41.0179, -52.0546)
  line L337 (41.0179, -52.0546) -> (43.0743, -58.1546)
  line L338 (43.0743, -58.1546) -> (42.2191, -58.1546)
  line L339 (42.2191, -58.1546) -> (41.6655, -56.4492)
  line L340 (41.6655, -56.4492) -> (39.3372, -56.4492)
  line L341 (39.3372, -56.4492) -> (38.7835, -58.1546)
  line L342 (38.7835, -58.1546) -> (37.963, -58.1546)
  line L343 (41.443, -55.7571) -> (40.4989, -52.8851)
  line L344 (40.4989, -52.8851) -> (39.5596, -55.7571)
  line L345 (39.5596, -55.7571) -> (41.443, -55.7571)
  line L346 (47.1525, -58.1546) -> (46.3814, -58.1546)
  line L347 (46.3814, -58.1546) -> (46.3814, -57.6504)
  spline S354 degree 2 poles (46.3814, -57.6504) (46.0254, -57.9618) (45.3878, -58.2832) (44.9923, -58.2832) knots 0 0 0 1 2 2 2
  spline S355 degree 2 poles (44.9923, -58.2832) (44.6957, -58.2832) (44.1668, -58.0854) (43.974, -57.8729) knots 0 0 0 1 2 2 2
  spline S356 degree 2 poles (43.974, -57.8729) (43.7763, -57.6603) (43.5588, -57.0127) (43.5588, -56.5481) knots 0 0 0 1 2 2 2
  line L348 (43.5588, -56.5481) -> (43.5588, -53.5772)
  line L349 (43.5588, -53.5772) -> (44.3299, -53.5772)
  line L350 (44.3299, -53.5772) -> (44.3299, -56.1872)
  spline S357 degree 2 poles (44.3299, -56.1872) (44.3299, -56.553) (44.3843, -57.0325) (44.4782, -57.2105) knots 0 0 0 1 2 2 2
  spline S358 degree 2 poles (44.4782, -57.2105) (44.5721, -57.3884) (44.8934, -57.5515) (45.195, -57.5515) knots 0 0 0 1 2 2 2
  spline S359 degree 2 poles (45.195, -57.5515) (45.4767, -57.5515) (46.1144, -57.2302) (46.3814, -56.9979) knots 0 0 0 1 2 2 2
  line L351 (46.3814, -56.9979) -> (46.3814, -53.5772)
  line L352 (46.3814, -53.5772) -> (47.1525, -53.5772)
  line L353 (47.1525, -53.5772) -> (47.1525, -58.1546)
  spline S360 degree 2 poles (49.6538, -58.2436) (49.026, -58.2436) (48.3191, -57.5268) (48.3191, -56.7507) knots 0 0 0 1 2 2 2
  line L354 (48.3191, -56.7507) -> (48.3191, -54.2148)
  line L355 (48.3191, -54.2148) -> (47.8001, -54.2148)
  line L356 (47.8001, -54.2148) -> (47.8001, -53.5772)
  line L357 (47.8001, -53.5772) -> (48.3191, -53.5772)
  line L358 (48.3191, -53.5772) -> (48.3191, -52.2622)
  line L359 (48.3191, -52.2622) -> (49.0903, -52.2622)
  line L360 (49.0903, -52.2622) -> (49.0903, -53.5772)
  line L361 (49.0903, -53.5772) -> (50.509, -53.5772)
  line L362 (50.509, -53.5772) -> (50.509, -54.2148)
  line L363 (50.509, -54.2148) -> (49.0903, -54.2148)
  line L364 (49.0903, -54.2148) -> (49.0903, -56.3948)
  spline S361 degree 2 poles (49.0903, -56.3948) (49.0903, -56.7409) (49.115, -57.1215) (49.199, -57.2846) knots 0 0 0 1 2 2 2
  spline S362 degree 2 poles (49.199, -57.2846) (49.2682, -57.428) (49.5797, -57.5713) (49.8466, -57.5713) knots 0 0 0 1 2 2 2
  spline S363 degree 2 poles (49.8466, -57.5713) (50.0344, -57.5713) (50.3854, -57.4576) (50.4645, -57.423) knots 0 0 0 1 2 2 2
  line L365 (50.4645, -57.423) -> (50.509, -57.423)
  line L366 (50.509, -57.423) -> (50.509, -58.1151)
  spline S364 degree 2 poles (50.509, -58.1151) (50.2915, -58.1744) (49.8466, -58.2436) (49.6538, -58.2436) knots 0 0 0 1 2 2 2
  spline S365 degree 2 poles (54.8393, -55.8659) (54.8393, -57.0226) (53.7271, -58.2832) (52.7977, -58.2832) knots 0 0 0 1 2 2 2
  spline S366 degree 2 poles (52.7977, -58.2832) (51.8437, -58.2832) (50.7512, -56.9831) (50.7512, -55.8659) knots 0 0 0 1 2 2 2
  spline S367 degree 2 poles (50.7512, -55.8659) (50.7512, -54.7191) (51.8783, -53.4486) (52.7977, -53.4486) knots 0 0 0 1 2 2 2
  spline S368 degree 2 poles (52.7977, -53.4486) (53.7271, -53.4486) (54.8393, -54.7141) (54.8393, -55.8659) knots 0 0 0 1 2 2 2
  spline S369 degree 2 poles (54.0434, -55.8659) (54.0434, -54.9761) (53.3959, -54.111) (52.7977, -54.111) knots 0 0 0 1 2 2 2
  spline S370 degree 2 poles (52.7977, -54.111) (52.1996, -54.111) (51.5471, -54.9761) (51.5471, -55.8659) knots 0 0 0 1 2 2 2
  spline S371 degree 2 poles (51.5471, -55.8659) (51.5471, -56.731) (52.1996, -57.6208) (52.7977, -57.6208) knots 0 0 0 1 2 2 2
  spline S372 degree 2 poles (52.7977, -57.6208) (53.3909, -57.6208) (54.0434, -56.7458) (54.0434, -55.8659) knots 0 0 0 1 2 2 2
  line L367 (60.8207, -58.1546) -> (60.8207, -55.505)
  spline S373 degree 2 poles (60.8207, -55.505) (60.8207, -55.1887) (60.7712, -54.6498) (60.6921, -54.5015) knots 0 0 0 1 2 2 2
  spline S374 degree 2 poles (60.6921, -54.5015) (60.613, -54.3384) (60.3115, -54.1802) (60.0495, -54.1802) knots 0 0 0 1 2 2 2
  spline S375 degree 2 poles (60.0495, -54.1802) (59.8122, -54.1802) (59.2685, -54.4719) (58.9818, -54.7487) knots 0 0 0 1 2 2 2
  spline S376 degree 2 poles (58.9818, -54.7487) (58.9867, -54.8179) (58.9966, -55.0107) (58.9966, -55.1392) knots 0 0 0 1 2 2 2
  line L368 (58.9966, -55.1392) -> (58.9966, -58.1546)
  line L369 (58.9966, -58.1546) -> (58.2254, -58.1546)
  line L370 (58.2254, -58.1546) -> (58.2254, -55.505)
  spline S377 degree 2 poles (58.2254, -55.505) (58.2254, -55.1887) (58.176, -54.6498) (58.0969, -54.5015) knots 0 0 0 1 2 2 2
  spline S378 degree 2 poles (58.0969, -54.5015) (58.0178, -54.3384) (57.7163, -54.1802) (57.4543, -54.1802) knots 0 0 0 1 2 2 2
  spline S379 degree 2 poles (57.4543, -54.1802) (57.2071, -54.1802) (56.6584, -54.4917) (56.4014, -54.7339) knots 0 0 0 1 2 2 2
  line L371 (56.4014, -54.7339) -> (56.4014, -58.1546)
  line L372 (56.4014, -58.1546) -> (55.6302, -58.1546)
  line L373 (55.6302, -58.1546) -> (55.6302, -53.5772)
  line L374 (55.6302, -53.5772) -> (56.4014, -53.5772)
  line L375 (56.4014, -53.5772) -> (56.4014, -54.0814)
  spline S380 degree 2 poles (56.4014, -54.0814) (56.7029, -53.7798) (57.2961, -53.4486) (57.652, -53.4486) knots 0 0 0 1 2 2 2
  spline S381 degree 2 poles (57.652, -53.4486) (58.0574, -53.4486) (58.6852, -53.8194) (58.8483, -54.2396) knots 0 0 0 1 2 2 2
  spline S382 degree 2 poles (58.8483, -54.2396) (59.1993, -53.849) (59.8617, -53.4486) (60.2472, -53.4486) knots 0 0 0 1 2 2 2
  spline S383 degree 2 poles (60.2472, -53.4486) (60.5438, -53.4486) (61.0283, -53.6315) (61.2062, -53.8391) knots 0 0 0 1 2 2 2
  spline S384 degree 2 poles (61.2062, -53.8391) (61.3891, -54.0468) (61.5918, -54.6696) (61.5918, -55.1392) knots 0 0 0 1 2 2 2
  line L376 (61.5918, -55.1392) -> (61.5918, -58.1546)
  line L377 (61.5918, -58.1546) -> (60.8207, -58.1546)
  spline S385 degree 2 poles (65.2251, -57.6702) (65.1312, -57.7394) (64.8148, -57.9866) (64.6665, -58.0607) knots 0 0 0 1 2 2 2
  spline S386 degree 2 poles (64.6665, -58.0607) (64.4639, -58.1695) (64.0832, -58.2832) (63.7372, -58.2832) knots 0 0 0 1 2 2 2
  spline S387 degree 2 poles (63.7372, -58.2832) (63.4554, -58.2832) (62.9463, -58.0706) (62.7535, -57.8778) knots 0 0 0 1 2 2 2
  spline S388 degree 2 poles (62.7535, -57.8778) (62.5706, -57.69) (62.3481, -57.1363) (62.3481, -56.8298) knots 0 0 0 1 2 2 2
  spline S389 degree 2 poles (62.3481, -56.8298) (62.3481, -56.3553) (62.7485, -55.683) (63.1835, -55.4902) knots 0 0 0 1 2 2 2
  spline S390 degree 2 poles (63.1835, -55.4902) (63.5691, -55.3122) (64.6171, -55.1788) (65.2251, -55.1442) knots 0 0 0 1 2 2 2
  line L378 (65.2251, -55.1442) -> (65.2251, -54.9959)
  spline S391 degree 2 poles (65.2251, -54.9959) (65.2251, -54.7289) (65.062, -54.3977) (64.9137, -54.3038) knots 0 0 0 1 2 2 2
  spline S392 degree 2 poles (64.9137, -54.3038) (64.7654, -54.2099) (64.3403, -54.1506) (64.1129, -54.1506) knots 0 0 0 1 2 2 2
  spline S393 degree 2 poles (64.1129, -54.1506) (63.8459, -54.1506) (63.1242, -54.3088) (62.7634, -54.462) knots 0 0 0 1 2 2 2
  line L379 (62.7634, -54.462) -> (62.7189, -54.462)
  line L380 (62.7189, -54.462) -> (62.7189, -53.676)
  spline S394 degree 2 poles (62.7189, -53.676) (62.9314, -53.6167) (63.7273, -53.4684) (64.1178, -53.4684) knots 0 0 0 1 2 2 2
  spline S395 degree 2 poles (64.1178, -53.4684) (64.5924, -53.4684) (65.24, -53.6167) (65.497, -53.8095) knots 0 0 0 1 2 2 2
  spline S396 degree 2 poles (65.497, -53.8095) (65.7491, -53.9973) (65.9963, -54.5955) (65.9963, -55.0255) knots 0 0 0 1 2 2 2
  line L381 (65.9963, -55.0255) -> (65.9963, -58.1546)
  line L382 (65.9963, -58.1546) -> (65.2251, -58.1546)
  line L383 (65.2251, -58.1546) -> (65.2251, -57.6702)
  line L384 (65.2251, -57.0276) -> (65.2251, -55.7571)
  spline S397 degree 2 poles (65.2251, -55.7571) (64.9483, -55.7819) (64.1129, -55.8659) (63.8509, -55.945) knots 0 0 0 1 2 2 2
  spline S398 degree 2 poles (63.8509, -55.945) (63.5444, -56.0389) (63.144, -56.4294) (63.144, -56.7755) knots 0 0 0 1 2 2 2
  spline S399 degree 2 poles (63.144, -56.7755) (63.144, -57.1709) (63.5889, -57.5713) (64.014, -57.5713) knots 0 0 0 1 2 2 2
  spline S400 degree 2 poles (64.014, -57.5713) (64.3749, -57.5713) (64.9681, -57.2599) (65.2251, -57.0276) knots 0 0 0 1 2 2 2
  spline S401 degree 2 poles (68.463, -58.2436) (67.8352, -58.2436) (67.1283, -57.5268) (67.1283, -56.7507) knots 0 0 0 1 2 2 2
  line L385 (67.1283, -56.7507) -> (67.1283, -54.2148)
  line L386 (67.1283, -54.2148) -> (66.6092, -54.2148)
  line L387 (66.6092, -54.2148) -> (66.6092, -53.5772)
  line L388 (66.6092, -53.5772) -> (67.1283, -53.5772)
  line L389 (67.1283, -53.5772) -> (67.1283, -52.2622)
  line L390 (67.1283, -52.2622) -> (67.8994, -52.2622)
  line L391 (67.8994, -52.2622) -> (67.8994, -53.5772)
  line L392 (67.8994, -53.5772) -> (69.3182, -53.5772)
  line L393 (69.3182, -53.5772) -> (69.3182, -54.2148)
  line L394 (69.3182, -54.2148) -> (67.8994, -54.2148)
  line L395 (67.8994, -54.2148) -> (67.8994, -56.3948)
  spline S402 degree 2 poles (67.8994, -56.3948) (67.8994, -56.7409) (67.9241, -57.1215) (68.0082, -57.2846) knots 0 0 0 1 2 2 2
  spline S403 degree 2 poles (68.0082, -57.2846) (68.0774, -57.428) (68.3888, -57.5713) (68.6558, -57.5713) knots 0 0 0 1 2 2 2
  spline S404 degree 2 poles (68.6558, -57.5713) (68.8436, -57.5713) (69.1946, -57.4576) (69.2737, -57.423) knots 0 0 0 1 2 2 2
  line L396 (69.2737, -57.423) -> (69.3182, -57.423)
  line L397 (69.3182, -57.423) -> (69.3182, -58.1151)
  spline S405 degree 2 poles (69.3182, -58.1151) (69.1006, -58.1744) (68.6558, -58.2436) (68.463, -58.2436) knots 0 0 0 1 2 2 2
  line L398 (70.6726, -58.1546) -> (69.9015, -58.1546)
  line L399 (69.9015, -58.1546) -> (69.9015, -53.5772)
  line L400 (69.9015, -53.5772) -> (70.6726, -53.5772)
  line L401 (70.6726, -53.5772) -> (70.6726, -58.1546)
  line L402 (70.727, -52.8159) -> (69.852, -52.8159)
  line L403 (69.852, -52.8159) -> (69.852, -52.0151)
  line L404 (69.852, -52.0151) -> (70.727, -52.0151)
  line L405 (70.727, -52.0151) -> (70.727, -52.8159)
  spline S406 degree 2 poles (73.6237, -58.2584) (73.1492, -58.2584) (72.3632, -57.9668) (72.0814, -57.6702) knots 0 0 0 1 2 2 2
  spline S407 degree 2 poles (72.0814, -57.6702) (71.7997, -57.3785) (71.4882, -56.4789) (71.4882, -55.8758) knots 0 0 0 1 2 2 2
  spline S408 degree 2 poles (71.4882, -55.8758) (71.4882, -55.2727) (71.8096, -54.3928) (72.0814, -54.0962) knots 0 0 0 1 2 2 2